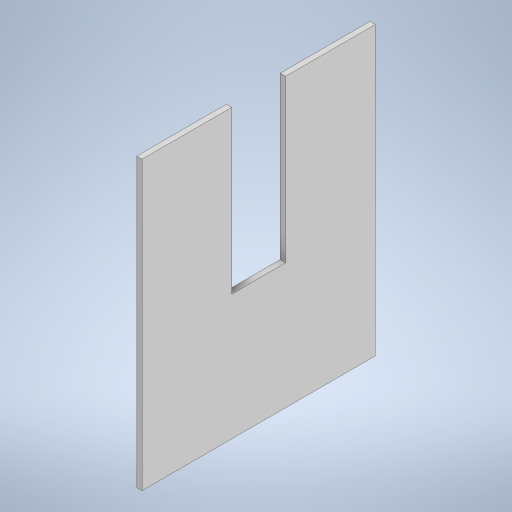
# Autodesk Inventor part: sadak
Saved by Autodesk Inventor 2023 (Build 270158000, 158)
## iProperties
Created: 2023-02-10
Part Number: sadak
Material: Generic
Document SubType Name: Modeling
Designer: deepa
Density: 1 g/cm^3
Appearance: Default
Author: deepa
Autodesk Inventor part; units mm, degrees
ref_plane "YZ Plane" through (0, 0, 0) normal (1, 0, 0) x (0, 1, 0)
ref_plane "XZ Plane" through (0, 0, 0) normal (0, 1, 0) x (-1, 0, 0)
ref_plane "XY Plane" through (0, 0, 0) normal (0, 0, 1) x (1, 0, 0)
sketch "Sketch1" plane through (0, 0, 0) normal (1, 0, 0) x (0, 1, 0)
  point P0 (0, 0)
sketch "Sketch2" plane through (0, 0, 0) normal (1, 0, 0) x (0, 1, 0)
  point P0 (0, 0)
sketch "Sketch3" plane through (0, 0, 0) normal (1, 0, 0) x (0, 1, 0)
  line L0 (0, 0) -> (0, 130)
  line L1 (0, 130) -> (120, 130)
  line L2 (120, 130) -> (160, 130)
  line L3 (160, 130) -> (160, 80)
  line L4 (160, 80) -> (70, 80)
  line L5 (70, 80) -> (70, 50)
  line L6 (70, 50) -> (160, 50)
  line L7 (160, 50) -> (160, 0)
  line L8 (160, 0) -> (0, 0)
  point P0 (120, 80)
  point P1 (120, 50)
  dimension "d0" = 130
  dimension "d1" = 120
  dimension "d2" = 40
  dimension "d3" = 50
  dimension "d4" = 90
  dimension "d5" = 30
  dimension "d6" = 90
  constraints: 18 end point, 5 perpendicular, 4 point on line, 1 vertical
  measures "d0" distance of L0.start L0.end
  measures "d1" distance of L0.end L1.end
  measures "d2" distance of L1.end L2.end
  measures "d3" distance of L2.end L3.end
  measures "d4" distance of L3.end L4.end
  measures "d5" distance of L4.end L5.end
  measures "d6" distance of L5.end L6.end
extrude "Extrusion1" add sketch "Sketch3" along normal blind 3
body "Solid1"
